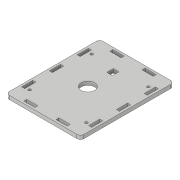
# Autodesk Inventor part: tapa2
Saved by Autodesk Inventor 2019 (Build 230136000, 136)
## iProperties
Created: 2018-09-20
Part Number: tapa2
Material: Genérico
Document SubType Name: Modeling
Designer: lmacia
Density: 1 g/cm^3
Appearance: Valor por defecto
Author: lmacia
Autodesk Inventor part; units mm, degrees
ref_plane "YZ Plane" through (0, 0, 0) normal (1, 0, 0) x (0, 1, 0)
ref_plane "XZ Plane" through (0, 0, 0) normal (0, 1, 0) x (-1, 0, 0)
ref_plane "XY Plane" through (0, 0, 0) normal (0, 0, 1) x (1, 0, 0)
sketch "Boceto1" plane through (0, 0, 0) normal (0, 1, 0) x (-1, 0, 0)
  line L0 (-31.7268, 34.9358) -> (-31.7268, -34.7768)
  line L1 (-28.9268, -37.5768) -> (25.401, -37.5769)
  line L2 (28.2018, -34.7802) -> (28.2019, 34.9339)
  line L3 (25.4109, 37.7268) -> (-28.9358, 37.7268)
  line L4 (-29.925, -4.425) -> (-29.925, 4.575)
  line L5 (-29.925, 4.575) -> (-29.85, 4.575)
  line L6 (-29.85, 4.575) -> (-27.6, 4.575)
  line L7 (-27.6, 4.575) -> (-27.525, 4.575)
  line L8 (-27.525, 4.575) -> (-27.525, -4.425)
  line L9 (-27.525, -4.425) -> (-27.6, -4.425)
  line L10 (-27.6, -4.425) -> (-29.85, -4.425)
  line L11 (-29.85, -4.425) -> (-29.925, -4.425)
  line L12 (26.4, -4.425) -> (26.325, -4.425)
  line L13 (26.325, -4.425) -> (24.075, -4.425)
  line L14 (24.075, -4.425) -> (24, -4.425)
  line L15 (24, -4.425) -> (24, 4.575)
  line L16 (24, 4.575) -> (24.075, 4.575)
  line L17 (24.075, 4.575) -> (26.325, 4.575)
  line L18 (26.325, 4.575) -> (26.4, 4.575)
  line L19 (26.4, 4.575) -> (26.4, -4.425)
  line L20 (26.325, 26.925) -> (26.4, 26.925)
  line L21 (26.4, 26.925) -> (26.4, 17.925)
  line L22 (26.4, 17.925) -> (26.325, 17.925)
  line L23 (26.325, 17.925) -> (24.075, 17.925)
  line L24 (24.075, 17.925) -> (24, 17.925)
  line L25 (24, 17.925) -> (24, 26.925)
  line L26 (24, 26.925) -> (24.075, 26.925)
  line L27 (24.075, 26.925) -> (26.325, 26.925)
  line L28 (-19.1813, -35.775) -> (-19.1813, -35.7)
  line L29 (-19.1813, -35.7) -> (-19.1813, -33.45)
  line L30 (-19.1813, -33.45) -> (-19.1813, -33.375)
  line L31 (-19.1813, -33.375) -> (-10.1813, -33.375)
  line L32 (-10.1813, -33.375) -> (-10.1813, -33.45)
  line L33 (-10.1813, -33.45) -> (-10.1813, -35.7)
  line L34 (-10.1813, -35.7) -> (-10.1813, -35.775)
  line L35 (-10.1813, -35.775) -> (-19.1813, -35.775)
  line L36 (6.6562, 33.525) -> (6.6562, 33.6)
  line L37 (6.6562, 33.6) -> (6.6562, 35.85)
  line L38 (6.6562, 35.85) -> (6.6562, 35.925)
  line L39 (6.6562, 35.925) -> (15.6562, 35.925)
  line L40 (15.6562, 35.925) -> (15.6562, 35.85)
  line L41 (15.6562, 35.85) -> (15.6562, 33.6)
  line L42 (15.6562, 33.6) -> (15.6562, 33.525)
  line L43 (15.6562, 33.525) -> (6.6562, 33.525)
  line L44 (-19.1813, 33.525) -> (-19.1813, 33.6)
  line L45 (-19.1813, 33.6) -> (-19.1813, 35.85)
  line L46 (-19.1813, 35.85) -> (-19.1813, 35.925)
  line L47 (-19.1813, 35.925) -> (-10.1813, 35.925)
  line L48 (-10.1813, 35.925) -> (-10.1813, 35.85)
  line L49 (-10.1813, 35.85) -> (-10.1813, 33.6)
  line L50 (-10.1813, 33.6) -> (-10.1813, 33.525)
  line L51 (-10.1813, 33.525) -> (-19.1813, 33.525)
  line L52 (24.075, -17.775) -> (26.325, -17.775)
  line L53 (26.325, -17.775) -> (26.4, -17.775)
  line L54 (26.4, -17.775) -> (26.4, -26.775)
  line L55 (26.4, -26.775) -> (26.325, -26.775)
  line L56 (26.325, -26.775) -> (24.075, -26.775)
  line L57 (24.075, -26.775) -> (24, -26.775)
  line L58 (24, -26.775) -> (24, -17.775)
  line L59 (24, -17.775) -> (24.075, -17.775)
  line L60 (6.6562, -35.775) -> (6.6562, -35.7)
  line L61 (6.6562, -35.7) -> (6.6562, -33.45)
  line L62 (6.6562, -33.45) -> (6.6562, -33.375)
  line L63 (6.6562, -33.375) -> (15.6562, -33.375)
  line L64 (15.6562, -33.375) -> (15.6562, -33.45)
  line L65 (15.6562, -33.45) -> (15.6562, -35.7)
  line L66 (15.6562, -35.7) -> (15.6562, -35.775)
  line L67 (15.6562, -35.775) -> (6.6562, -35.775)
  line L68 (-27.6, -26.775) -> (-29.85, -26.775)
  line L69 (-29.85, -26.775) -> (-29.925, -26.775)
  line L70 (-29.925, -26.775) -> (-29.925, -17.775)
  line L71 (-29.925, -17.775) -> (-29.85, -17.775)
  line L72 (-29.85, -17.775) -> (-27.6, -17.775)
  line L73 (-27.6, -17.775) -> (-27.525, -17.775)
  line L74 (-27.525, -17.775) -> (-27.525, -26.775)
  line L75 (-27.525, -26.775) -> (-27.6, -26.775)
  line L76 (-27.525, 26.925) -> (-27.525, 17.925)
  line L77 (-27.525, 17.925) -> (-27.6, 17.925)
  line L78 (-27.6, 17.925) -> (-29.85, 17.925)
  line L79 (-29.85, 17.925) -> (-29.925, 17.925)
  line L80 (-29.925, 17.925) -> (-29.925, 26.925)
  line L81 (-29.925, 26.925) -> (-29.85, 26.925)
  line L82 (-29.85, 26.925) -> (-27.6, 26.925)
  line L83 (-27.6, 26.925) -> (-27.525, 26.925)
  line L84 (-2.25, -17.475) -> (2.25, -17.475)
  line L85 (2.25, -17.475) -> (2.25, -22.725)
  line L86 (2.25, -22.725) -> (-2.25, -22.725)
  line L87 (-2.25, -22.725) -> (-2.25, -17.475)
  circle A0 centre (-24.6, 25.8) radius 1.05
  circle A1 centre (21.075, 25.8) radius 1.05
  circle A2 centre (0, 0) radius 5.4375
  arc A3 (-31.7268, -34.7768) -> (-28.9268, -37.5768) centre (-28.9268, -34.7768) ccw
  arc A4 (-28.9358, 37.7268) -> (-31.7268, 34.9358) centre (-28.9358, 34.9358) ccw
  arc A5 (25.401, -37.5769) -> (28.2018, -34.7802) centre (25.4018, -34.7769) ccw
  arc A6 (28.2019, 34.9339) -> (25.4109, 37.7268) centre (25.4108, 34.9357) ccw
  circle A7 centre (-24.6, -24.075) radius 1.05
  circle A8 centre (21.075, -24.075) radius 1.05
  line L88 (15.6562, 35.925) -> (6.6562, 35.925)
  line L89 (6.6562, 35.925) -> (6.6562, 33.525)
  line L90 (6.6562, 33.525) -> (15.6562, 33.525)
  line L91 (15.6562, 33.525) -> (15.6562, 35.925)
  line L92 (26.4, 26.925) -> (24, 26.925)
  line L93 (24, 26.925) -> (24, 17.925)
  line L94 (24, 17.925) -> (26.4, 17.925)
  line L95 (26.4, 17.925) -> (26.4, 26.925)
  line L96 (26.4, 4.575) -> (24, 4.575)
  line L97 (24, 4.575) -> (24, -4.425)
  line L98 (24, -4.425) -> (26.4, -4.425)
  line L99 (26.4, -4.425) -> (26.4, 4.575)
  line L100 (26.4, -17.775) -> (24, -17.775)
  line L101 (24, -17.775) -> (24, -26.775)
  line L102 (24, -26.775) -> (26.4, -26.775)
  line L103 (26.4, -26.775) -> (26.4, -17.775)
  line L104 (15.6562, -33.375) -> (6.6562, -33.375)
  line L105 (6.6562, -33.375) -> (6.6562, -35.775)
  line L106 (6.6562, -35.775) -> (15.6562, -35.775)
  line L107 (15.6562, -35.775) -> (15.6562, -33.375)
  line L108 (-10.1813, -33.375) -> (-19.1813, -33.375)
  line L109 (-19.1813, -33.375) -> (-19.1813, -35.775)
  line L110 (-19.1813, -35.775) -> (-10.1813, -35.775)
  line L111 (-10.1813, -35.775) -> (-10.1813, -33.375)
  line L112 (-27.525, -26.775) -> (-29.925, -26.775)
  line L113 (-29.925, -26.775) -> (-29.925, -17.775)
  line L114 (-29.925, -17.775) -> (-27.525, -17.775)
  line L115 (-27.525, -17.775) -> (-27.525, -26.775)
  line L116 (-27.525, -4.425) -> (-29.925, -4.425)
  line L117 (-29.925, -4.425) -> (-29.925, 4.575)
  line L118 (-29.925, 4.575) -> (-27.525, 4.575)
  line L119 (-27.525, 4.575) -> (-27.525, -4.425)
  line L120 (-27.525, 17.925) -> (-29.925, 17.925)
  line L121 (-29.925, 17.925) -> (-29.925, 26.925)
  line L122 (-29.925, 26.925) -> (-27.525, 26.925)
  line L123 (-27.525, 26.925) -> (-27.525, 17.925)
  line L124 (-19.1813, 35.925) -> (-10.1813, 35.925)
  line L125 (-10.1813, 35.925) -> (-10.1813, 33.525)
  line L126 (-10.1813, 33.525) -> (-19.1813, 33.525)
  line L127 (-19.1813, 33.525) -> (-19.1813, 35.925)
  line L128 (2.25, -17.475) -> (-2.25, -17.475)
  line L129 (-2.25, -17.475) -> (-2.25, -22.725)
  line L130 (-2.25, -22.725) -> (2.25, -22.725)
  line L131 (2.25, -22.725) -> (2.25, -17.475)
  constraints: 264 end point, 22 parallel, 11 horizontal, 11 perpendicular, 9 centre point, 8 point on circle
extrude "Extrusión1" add sketch "Boceto1" along normal blind 3
